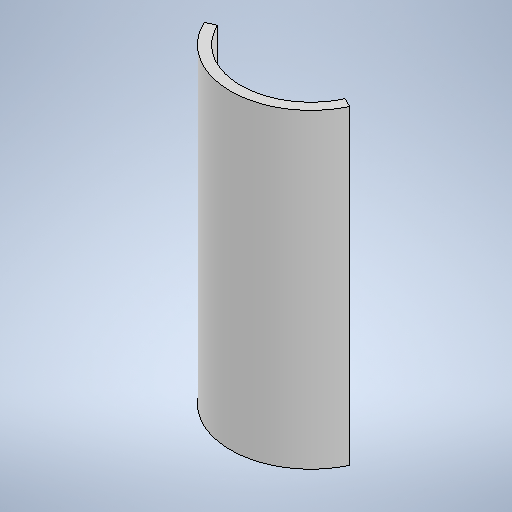
# Autodesk Inventor part: NVPH-303 second tube half
Saved by Autodesk Inventor 2025.1 (Build 291241020, 241B)
## iProperties
Created: 2024-12-03
Part Number: NVPH-303 second tube half
Material: Generic
Document SubType Name: Modeling
Designer: user
Density: 1 g/cm^3
Appearance: Default
Author: user
Autodesk Inventor part; units mm, degrees
ref_plane "YZ Plane" through (0, 0, 0) normal (1, 0, 0) x (0, 1, 0)
ref_plane "XZ Plane" through (0, 0, 0) normal (0, 1, 0) x (-1, 0, 0)
ref_plane "XY Plane" through (0, 0, 0) normal (0, 0, 1) x (1, 0, 0)
sketch "Sketch1" plane through (0, 0, 0) normal (0, 0, 1) x (1, 0, 0)
  circle A0 centre (0, 0) radius 70
  circle A1 centre (0, 0) radius 80
  dimension "d6" = 10
  dimension "d11" = 160
  constraints: 2 centre point, 2 coincident
  measures "d6" radial gap between concentric circles of A0 A1
  measures "d11" diameter of A1
extrude "Extrusion1" add sketch "Sketch1" along normal blind 310
sketch "Sketch5" plane through (0, 0, 0) normal (0, 0, 1) x (1, 0, 0)
  circle A0 centre (0, 0) radius 80 projected
  circle A1 centre (0, 0) radius 70 projected
  line L0 (0, 0) -> (-72.5046, -33.8095)
  line L1 (0, 0) -> (72.5046, -33.8095)
  line L2 (0, 0) -> (0, -80) construction
  point P0 (63.4415, -29.5833)
  point P1 (-63.4415, -29.5833)
  dimension "d8" = 130
  constraints: 6 end point, 3 point on circle, 1 vertical, 1 other
  measures "d8" angle of L1 L0
extrude "Extrusion3" cut sketch "Sketch5" along normal through all contours A0 L1 A1 L0 picked at (76.3447, 4.1316)
body "Solid1"
